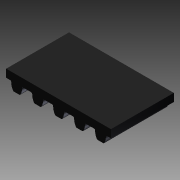
# Autodesk Inventor part: 5MR-900-15
Saved by Autodesk Inventor 2011 (Build 150239000, 239)
## iProperties
Category: Miscellaneous
Company: Autodesk Inc.
Created: 2008-12-31
Part Number: 5MR-900-15
Document SubType Name: Modeling
Designer: Autodesk Inc.
Density: 1 g/cm^3
Catalog Web Link: http://www.gates.com/catalogs/file_display.cfm?file=SynchronousBelts.pdf&thisPath=gates\catalogs
Description: PowerGrip GT2 long-length belting, 5mm pitch
Vendor: Gates Corporation
Author: Autodesk Inc.
Autodesk Inventor part; units mm, degrees
ref_plane "YZ Plane" through (0, 0, 0) normal (1, 0, 0) x (0, 1, 0)
ref_plane "XZ Plane" through (0, 0, 0) normal (0, 1, 0) x (-1, 0, 0)
ref_plane "XY Plane" through (0, 0, 0) normal (0, 0, 1) x (1, 0, 0)
sketch "Sketch1" plane through (0, 0, 0) normal (0, 0, 1) x (1, 0, 0)
  line L0 (-14.2973, 4.3336) -> (-13.3453, 4.3336)
  line L1 (-18.3453, 6.2132) -> (6.6546, 6.2132)
  arc A0 (-14.971, 2.5331) -> (-14.5513, 3.9796) centre (-17.2541, 3.9796) ccw
  arc A1 (-17.1394, 3.9796) -> (-16.7197, 2.5331) centre (-14.4366, 3.9796) ccw
  arc A2 (-15.207, 2.4032) -> (-14.971, 2.5331) centre (-15.207, 2.6826) ccw
  arc A3 (-16.7197, 2.5331) -> (-16.4837, 2.4032) centre (-16.4837, 2.6826) ccw
  line L2 (-15.8453, 2.4032) -> (-15.207, 2.4032)
  line L3 (-15.8453, 2.4032) -> (-16.4837, 2.4032)
  arc A4 (-14.2973, 4.3336) -> (-14.5513, 4.0796) centre (-14.2973, 4.0796) ccw
  arc A5 (-17.1394, 4.0796) -> (-17.3934, 4.3336) centre (-17.3934, 4.0796) ccw
  line L4 (-18.3453, 4.3336) -> (-18.3453, 6.2132)
  line L5 (-14.5513, 3.9796) -> (-14.5513, 4.0796)
  line L6 (-17.3934, 4.3336) -> (-18.3453, 4.3336)
  line L7 (-17.1394, 3.9796) -> (-17.1394, 4.0796)
  arc A6 (5.029, 2.5331) -> (5.4487, 3.9796) centre (2.7459, 3.9796) ccw
  arc A7 (2.8606, 3.9796) -> (3.2803, 2.5331) centre (5.5634, 3.9796) ccw
  arc A8 (0.029, 2.5331) -> (0.4487, 3.9796) centre (-2.2541, 3.9796) ccw
  arc A9 (-2.1394, 3.9796) -> (-1.7197, 2.5331) centre (0.5634, 3.9796) ccw
  arc A10 (-4.971, 2.5331) -> (-4.5513, 3.9796) centre (-7.2541, 3.9796) ccw
  arc A11 (-7.1394, 3.9796) -> (-6.7197, 2.5331) centre (-4.4366, 3.9796) ccw
  arc A12 (-9.971, 2.5331) -> (-9.5513, 3.9796) centre (-12.2541, 3.9796) ccw
  arc A13 (-12.1394, 3.9796) -> (-11.7197, 2.5331) centre (-9.4366, 3.9796) ccw
  arc A14 (-10.207, 2.4032) -> (-9.971, 2.5331) centre (-10.207, 2.6826) ccw
  line L8 (-10.8453, 2.4032) -> (-10.207, 2.4032)
  arc A15 (-11.7197, 2.5331) -> (-11.4837, 2.4032) centre (-11.4837, 2.6826) ccw
  line L9 (-10.8453, 2.4032) -> (-11.4837, 2.4032)
  arc A16 (-5.207, 2.4032) -> (-4.971, 2.5331) centre (-5.207, 2.6826) ccw
  line L10 (-5.8453, 2.4032) -> (-5.207, 2.4032)
  arc A17 (-6.7197, 2.5331) -> (-6.4837, 2.4032) centre (-6.4837, 2.6826) ccw
  line L11 (-5.8453, 2.4032) -> (-6.4837, 2.4032)
  arc A18 (-0.207, 2.4032) -> (0.029, 2.5331) centre (-0.207, 2.6826) ccw
  line L12 (-0.8454, 2.4032) -> (-0.207, 2.4032)
  arc A19 (-1.7197, 2.5331) -> (-1.4837, 2.4032) centre (-1.4837, 2.6826) ccw
  line L13 (-0.8454, 2.4032) -> (-1.4837, 2.4032)
  arc A20 (4.793, 2.4032) -> (5.029, 2.5331) centre (4.793, 2.6826) ccw
  line L14 (4.1546, 2.4032) -> (4.793, 2.4032)
  arc A21 (3.2803, 2.5331) -> (3.5163, 2.4032) centre (3.5163, 2.6826) ccw
  line L15 (4.1546, 2.4032) -> (3.5163, 2.4032)
  line L16 (-2.3934, 4.3336) -> (-3.3454, 4.3336)
  line L17 (-9.2973, 4.3336) -> (-8.3453, 4.3336)
  line L18 (-9.5513, 3.9796) -> (-9.5513, 4.0796)
  arc A22 (-9.2973, 4.3336) -> (-9.5513, 4.0796) centre (-9.2973, 4.0796) ccw
  line L19 (-12.1394, 3.9796) -> (-12.1394, 4.0796)
  arc A23 (-12.1394, 4.0796) -> (-12.3934, 4.3336) centre (-12.3934, 4.0796) ccw
  line L20 (-12.3934, 4.3336) -> (-13.3453, 4.3336)
  line L21 (-4.5513, 3.9796) -> (-4.5513, 4.0796)
  arc A24 (-4.2973, 4.3336) -> (-4.5513, 4.0796) centre (-4.2973, 4.0796) ccw
  line L22 (-4.2973, 4.3336) -> (-3.3454, 4.3336)
  line L23 (-7.1394, 3.9796) -> (-7.1394, 4.0796)
  arc A25 (-7.1394, 4.0796) -> (-7.3934, 4.3336) centre (-7.3934, 4.0796) ccw
  line L24 (-7.3934, 4.3336) -> (-8.3453, 4.3336)
  line L25 (2.6066, 4.3336) -> (1.6546, 4.3336)
  line L26 (0.4487, 3.9796) -> (0.4487, 4.0796)
  arc A26 (0.7027, 4.3336) -> (0.4487, 4.0796) centre (0.7027, 4.0796) ccw
  line L27 (0.7027, 4.3336) -> (1.6546, 4.3336)
  line L28 (-2.1394, 3.9796) -> (-2.1394, 4.0796)
  arc A27 (-2.1394, 4.0796) -> (-2.3934, 4.3336) centre (-2.3934, 4.0796) ccw
  line L29 (5.4487, 3.9796) -> (5.4487, 4.0796)
  arc A28 (5.7027, 4.3336) -> (5.4487, 4.0796) centre (5.7027, 4.0796) ccw
  line L30 (5.7027, 4.3336) -> (6.6546, 4.3336)
  line L31 (2.8606, 3.9796) -> (2.8606, 4.0796)
  arc A29 (2.8606, 4.0796) -> (2.6066, 4.3336) centre (2.6066, 4.0796) ccw
  line L32 (6.6546, 4.3336) -> (6.6546, 6.2132)
  line L33 (6.0839, 4.3336) -> (6.6546, 4.3336)
  dimension "d2" = 5
  dimension "d3" = 3.81
  dimension "d4" = 1.9304
  constraints: 68 end point, 60 point on circle, 30 centre point, 1 point on line
  measures "d2" distance of L8.start L2.start
  measures "d3" distance between parallel lines of L3 L1
  measures "d4" distance between parallel lines of L14 L30
extrude "Extrusion1" add sketch "Sketch1" along normal blind 15
body "Solid1"
